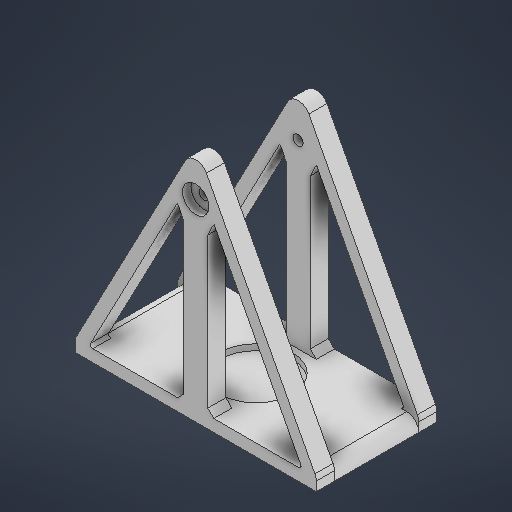
# Autodesk Inventor part: EncaixeBase
Saved by Autodesk Inventor 2026 (Build 300175050, 175E)
## iProperties
Created: 2025-03-17
Part Number: EncaixeBase
Material: Genérico
Document SubType Name: Modeling
Designer: Ian
Density: 1 g/cm^3
Appearance: Padrão
Author: Ian
Autodesk Inventor part; units mm, degrees
ref_plane "YZ Plane" through (0, 0, 0) normal (1, 0, 0) x (0, 1, 0)
ref_plane "XZ Plane" through (0, 0, 0) normal (0, 1, 0) x (-1, 0, 0)
ref_plane "XY Plane" through (0, 0, 0) normal (0, 0, 1) x (1, 0, 0)
sketch "Esboço1" plane through (0, 0, 0) normal (0, 0, 1) x (1, 0, 0)
  line L0 (-100, 5) -> (100, 5)
  line L1 (100, 5) -> (100, -5)
  line L2 (100, -5) -> (-100, -5)
  line L3 (-100, -5) -> (-100, 5)
  line L4 (-100, 5) -> (100, -5) construction
  line L5 (100, 5) -> (-100, -5) construction
  point P0 (0, 0)
  dimension "d0" = 200
  dimension "d1" = 10
  constraints: 12 end point, 2 midpoint, 2 parallel, 1 horizontal, 1 perpendicular
  measures "d0" distance of L1.end L2.end
  measures "d1" distance of L0.end L1.end
extrude "Extrusão1" add sketch "Esboço1" along normal blind 100
sketch "Esboço2" plane through (0, 0, 100) normal (0, 0, 1) x (1, 0, 0)
  line L0 (100, 5) -> (-100, 5) projected
  line L1 (100, 5) -> (-100, 5) projected
  line L2 (-100, -5) -> (100, -5) projected
  line L3 (0, -5) -> (0, 195) construction
  line L4 (0, 195) -> (-100, 5)
  line L5 (0, 195) -> (100, 5)
  point P0 (0, 0)
  point P1 (0, 5)
  dimension "d20" = 200
  constraints: 6 end point, 2 midpoint, 1 vertical
  measures "d20" distance of L3.start L3.end
extrude "Extrusão2" add sketch "Esboço2" against normal blind 15
sketch "Esboço3" plane through (0, 0, 0) normal (0, 0, -1) x (-1, 0, 0)
  line L0 (-100, 5) -> (100, 5)
  line L1 (100, -5) -> (-100, -5) projected
  line L2 (0, -5) -> (0, 195) construction
  line L3 (-100, -5) -> (-100, 5) projected
  line L4 (0, 195) -> (-100, 5)
  line L5 (0, 195) -> (100, 5)
  point P0 (0, 0)
  dimension "d21" = 200
  constraints: 8 end point, 1 midpoint, 1 vertical
  measures "d21" distance of L2.start L2.end
extrude "Extrusão3" add sketch "Esboço3" against normal blind 15
sketch "Esboço4" plane through (0, 0, 100) normal (0, 0, 1) x (1, 0, 0)
  circle A0 centre (0, 155) radius 4.25
  line L0 (-100, -5) -> (100, -5) projected
  line L1 (100, 5) -> (0, 195) projected
  line L2 (0, 195) -> (0, -5) construction
  point P0 (0, 0)
  dimension "d13" = 8.5
  dimension "d22" = 160
  constraints: 2 end point, 2 vertical, 1 centre point, 1 midpoint
  measures "d13" diameter of A0
  measures "d22" distance of L2.end A0.centre
extrude "Extrusão4" cut sketch "Esboço4" against normal through all
fillet "Arredondamento3" radius 10 2 edges at (0, 195, 92.5) (0, 195, 7.5)
sketch "Esboço5" plane through (0, 0, 100) normal (0, 0, 1) x (1, 0, 0)
  circle A0 centre (0, 155) radius 4.25 projected
  circle A1 centre (0, 155) radius 10.975
  point P0 (0, 0)
  dimension "d25" = 21.95
  constraints: 1 centre point, 1 coincident
  measures "d25" diameter of A1
extrude "Extrusão5" cut sketch "Esboço5" against normal blind 7
sketch "Esboço6" plane through (0, 0, 0) normal (0, 0, -1) x (-1, 0, 0)
  circle A0 centre (0, 155) radius 4.25 projected
  circle A1 centre (0, 155) radius 10.975
  point P0 (0, 0)
  dimension "d28" = 21.95
  constraints: 1 centre point, 1 coincident
  measures "d28" diameter of A1
extrude "Extrusão6" cut sketch "Esboço6" against normal blind 7
sketch "Esboço7" plane through (0, 0, 0) normal (0, 0, -1) x (-1, 0, 0)
  circle A0 centre (0, 155) radius 10.975 projected
  circle A1 centre (0, 155) radius 18.6299
  line L0 (100, 5) -> (8.8492, 178.1866) projected
  line L1 (15.3264, 144.4089) -> (88.6995, 5)
  line L2 (100, 5) -> (-100, 5) projected
  line L3 (88.6995, 5) -> (-88.6995, 5)
  line L4 (-15.3264, 144.4089) -> (-88.6995, 5)
  line L5 (100, 5) -> (8.8492, 178.1866) projected
  line L6 (-8.8492, 178.1866) -> (-100, 5) projected
  circle A2 centre (0, 155) radius 4.25 projected
  line L7 (0, 155) -> (0, -5.3042)
  line L8 (10, 139.2815) -> (10, 5)
  line L9 (-10, 139.2815) -> (-10, 5)
  point P0 (0, 0)
  point P1 (-10.946, 174.2026)
  point P2 (10.946, 174.2026)
  dimension "d31" = 10
  dimension "d32" = 10
  dimension "d39" = 10
  dimension "d40" = 10
  constraints: 12 end point, 4 parallel, 4 point on circle, 4 point on line, 2 vertical, 1 centre point, 1 coincident, 1 perpendicular, 1 tangent, 1 other
  measures "d31" distance between parallel lines of L0 L1
  measures "d32" distance between parallel lines of L6 L4
  measures "d39" distance between parallel lines of L8 L7
  measures "d40" distance between parallel lines of L7 L9
extrude "Extrusão7" cut sketch "Esboço7" against normal through all contours A1 L9 L2 L4 | A1 L1 L2 L8
sketch "Esboço8" plane through (100, 5, 85) normal (0, 1, 0) x (1, 0, 0)
  line L0 (-200, 85) -> (0, 85) projected
  line L1 (-108.8492, -15) -> (-200, -15) projected
  line L2 (0, 85) -> (-200, 85)
  line L3 (-200, 85) -> (-200, -15)
  line L4 (-200, -15) -> (0, -15)
  line L5 (0, -15) -> (0, 85)
  line L6 (0, 35) -> (-200, 35) construction
  line L7 (-100, -15) -> (-100, 85) construction
  line L8 (-91.1508, 0) -> (0, 0) projected
  circle A0 centre (-100, 35) radius 30
  point P0 (-110.946, -15)
  dimension "d35" = 60
  constraints: 12 end point, 4 midpoint, 2 parallel, 2 perpendicular, 1 centre point, 1 horizontal
  measures "d35" diameter of A0
extrude "Extrusão8" cut sketch "Esboço8" against normal blind 5 contours A0
chamfer "Chanfro1" distance 5 angle 45 8 edges at (-10, 139.2815, 92.5) (10, 139.2815, 92.5) (10, 139.2815, 7.5) (-10, 139.2815, 7.5) (10, 5, 7.5) (-10, 5, 7.5) (-10, 5, 92.5) (10, 5, 92.5)
fillet "Arredondamento5" radius 2 4 edges at (88.6995, 5, 92.5) (-88.6995, 5, 92.5) (88.6995, 5, 7.5) (-88.6995, 5, 7.5)
fillet "Arredondamento6" radius 10 2 edges at (-100, 5, 50) (100, 5, 50)
fillet "Arredondamento7" radius 10 4 edges at (100, 5, 92.5) (100, 5, 7.5) (-100, 5, 92.5) (-100, 5, 7.5)
